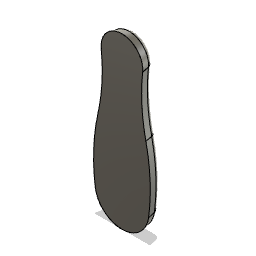
Robot_assembly (Autodesk Fusion 360 archive; units mm, degrees)
design "RBT_LINK2"
Autodesk Fusion 360 part; units mm, degrees
sketch "Sketch2" plane through (0, 0, 0) normal (0, 0, 1) x (1, 0, 0)
  arc A0 (29.8304, 196.8149) -> (35.2531, 100) centre (328.1348, 164.9639) ccw
  arc A1 (39.6352, -5.3902) -> (35.2531, 100) centre (-257.6286, 35.0361) ccw
  line L0 (0, 200) -> (0, 0) construction
  arc A2 (-35.2531, 100) -> (-29.8304, 196.8149) centre (-328.1348, 164.9639) ccw
  arc A3 (-35.2531, 100) -> (-39.6352, -5.3902) centre (257.6286, 35.0361) ccw
  arc A4 (29.8304, 196.8149) -> (-29.8304, 196.8149) centre (0, 200) ccw
  arc A5 (-39.6352, -5.3902) -> (39.6352, -5.3902) centre (0, 0) ccw
  dimension "d5" = 80
  dimension "d6" = 60
  dimension "d7" = 200
  dimension "d8" = 100
  dimension "d9" = 300
  constraint coincident L0.end A5.centre
  constraint vertical L0.end L0.start
  constraint tangent A0 A1
  constraint tangent A0 A4
  constraint tangent A1 A5
  constraint equal A0 A1
  constraint coincident L0.start A4.centre
  constraint symmetric A0.start L0 A2.end
  constraint symmetric A0.end L0 A2.start
  constraint symmetric A0 L0 A2
  constraint symmetric A1.start L0 A3.end
  constraint symmetric A1 L0 A3
  measures "d5" diameter of A5
  measures "d6" diameter of A4
  measures "d7" distance of L0.end L0.start
  measures "d8" vertical distance of L0.end A0.end
  measures "d9" radius of A0
extrude "Extrude1" add sketch "Sketch2" along normal blind 20
draft "Draft1" angle 12 neutral plane through (0, 0, 0) pull (0, 0, -1) 6 faces at (33.1008, 110.6047, 6.6667) (-29.95, 198.2683, 6.6667) (-28.3505, 153.5916, 6.6667) (-39.4474, 76.8197, 6.6667) (18.4195, -35.5067, 13.3333) (42.2994, 41.6114, 6.6667)
fillet "Fillet1" radius 10 6 edges at (-28.6043, 148.1869, 0) (-42.1125, 47.499, 0) (0, -40, 0) (42.1125, 47.499, 0) (28.6043, 148.1869, 0) (0, 230, 0)
shell "Shell4" [rolled back] inner thickness 3
ref_plane "WorkPlane1" through (0, 98.0755, 15) normal (0, 0, 1) x (1, 0, 0)
sketch "Sketch3" plane through (0, 98.0755, 15) normal (0, 0, 1) x (1, 0, 0)
  line L0 (-10, 90) -> (10, 90)
  line L1 (-10, 40) -> (10, 40)
  line L2 (-20, -20) -> (10, -20)
  line L3 (-20, -70) -> (20, -70)
  line L4 (-10, -113.3333) -> (9.4128, -113.3333)
  line L5 (-10, 20) -> (-10, -10)
  line L6 (10, 20) -> (10, -10)
  constraint horizontal L0
  constraint horizontal L1
  constraint horizontal L2
  constraint horizontal L3
  constraint horizontal L4
  constraint perpendicular L2 L5
  constraint vertical L6
web "Web1" [rolled back] thickness 2
sketch "Sketch4" plane through (0, 0, 0) normal (0, 1, 0) x (1, 0, 0)
  line L0 (-9, -3) -> (9, -15)
rib "Rib1" [rolled back] thickness 2 thickness 2

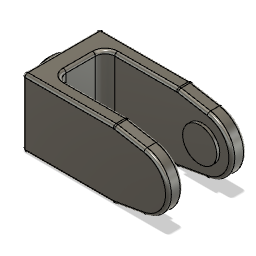
design "RBT_LINK4"
Autodesk Fusion 360 part; units mm, degrees
sketch "Sketch1" plane through (0, 0, 0) normal (0, 0, 1) x (1, 0, 0)
  line L0 (0, 0) -> (94.2683, 0)
  line L1 (94.2683, 0) -> (125.2094, 5.4558)
  arc A0 (125.2094, 5.4558) -> (125.2094, 64.5442) centre (120, 35) ccw
  line L2 (125.2094, 64.5442) -> (94.2683, 70)
  line L3 (94.2683, 70) -> (0, 70)
  line L4 (0, 70) -> (0, 0)
  dimension "d1" = 70
  dimension "d2" = 30
  dimension "d3" = 170
  dimension "d4" = 120
  constraint coincident L0.start L4.end
  constraint horizontal L0
  constraint tangent L1 A0
  constraint tangent A0 L2
  constraint horizontal L3
  constraint perpendicular L0 L4
  constraint equal L1 L2
  constraint equal L0 L3
  measures "d1" distance of L0 L3
  measures "d2" radius of A0
  measures "d3" angle of L0 L1
  measures "d4" horizontal distance of L0.start A0.centre
extrude "Extrude1" add sketch "Sketch1" along normal mid plane 80
sketch "Sketch2" plane through (0, 70, 0) normal (0, 1, 0) x (-1, 0, 0)
  line L0 (0, -40) -> (0, 40)
  line L1 (0, 40) -> (-94.2683, 40)
  line L2 (-94.2683, 40) -> (-94.2683, -40)
  line L3 (-94.2683, -40) -> (0, -40)
  line L4 (-20, -25) -> (-190, -25)
  line L5 (-190, -25) -> (-190, 25)
  line L6 (-190, 25) -> (-20, 25)
  line L7 (-20, 25) -> (-20, -25)
  dimension "d7" = 15
  dimension "d8" = 15
  dimension "d9" = 20
  dimension "d10" = 170
  constraint horizontal L4
  constraint vertical L5
  constraint horizontal L6
  constraint vertical L7
  measures "d7" distance of L3 L4
  measures "d8" distance of L1 L6
  measures "d9" distance of L0 L7
  measures "d10" distance of L5.end L6.end
extrude "Extrude2" cut sketch "Sketch2" against normal through all contours L2 L4 L5 L6 | L2 L4 L6 L7
sketch "Sketch3" plane through (0, 0, -25) normal (0, 0, 1) x (1, 0, 0)
  line L0 (20, 0) -> (94.2683, 0)
  line L1 (94.2683, 0) -> (125.2094, 5.4558)
  arc A0 (125.2094, 5.4558) -> (125.2094, 64.5442) centre (120, 35) ccw
  line L2 (125.2094, 64.5442) -> (94.2683, 70)
  line L3 (94.2683, 70) -> (20, 70)
  line L4 (20, 70) -> (20, 0)
  circle A1 centre (120, 35) radius 17.5
  dimension "d12" = 35
  constraint concentric A0 A1
  measures "d12" diameter of A1
extrude "Extrude3" add sketch "Sketch3" along normal blind 3 contours A1
mirror "Mirror1" about plane through (0, 0, 0) normal (0, 0, 1) of "Extrude3"
sketch "Sketch4" plane through (0, 0, 0) normal (-1, 0, 0) x (0, 0, 1)
  line L0 (-40, 0) -> (40, 0)
  line L1 (40, 0) -> (40, 70)
  line L2 (40, 70) -> (-40, 70)
  line L3 (-40, 70) -> (-40, 0)
  circle A0 centre (0, 35) radius 25
  line L4 (0, 35) -> (-40, 35) construction
  line L5 (0, 35) -> (0, 0) construction
  dimension "d16" = 50
  constraint coincident A0.centre L4.start
  constraint midpoint L3 L4.end
  constraint perpendicular L3 L4
  constraint coincident L5.end origin
  constraint perpendicular L0 L5
  measures "d16" diameter of A0
extrude "Extrude4" add sketch "Sketch4" along normal blind 10 contours A0
sketch "Sketch5" plane through (-10, 0, 0) normal (-1, 0, 0) x (0, 0, 1)
  circle A0 centre (0, 35) radius 25
  circle A1 centre (0, 35) radius 22
  dimension "d19" = -3
extrude "Extrude5" add sketch "Sketch5" along normal blind 3 contours A1
fillet "Fillet1" radius 10 6 edges at (20, 35, 25) (20, 35, -25) (94.2683, 70, 32.5) (94.2683, 70, -32.5) (94.2683, 0, 32.5) (94.2683, 0, -32.5)
fillet "Fillet2" radius 3 39 edges at (46.6967, 0, 40) (94.2649, 0.0381, 40) (110.1696, 2.8038, 40) (150, 35, 40) (110.1696, 67.1962, 40) (94.2649, 69.9619, 40) (46.6967, 70, 40) (46.6967, 70, -40) (94.2649, 69.9619, -40) (110.1696, 67.1962, -40) (150, 35, -40) (110.1696, 2.8038, -40) (94.2649, 0.0381, -40) (46.6967, 0, -40) (0, 70, 0) (0, 35, 40) (0, 35, -40) (0, 0, 0) (0, 44.0404, -23.3082) (22.9289, 70, 22.0711) (20, 70, 0) (22.9289, 70, -22.0711) (61.6967, 70, -25) (94.2649, 69.9619, -25) (110.1696, 67.1962, -25) (150, 35, -25) (110.1696, 2.8038, -25) (94.2649, 0.0381, -25) (61.6967, 0, -25) (22.9289, 0, -22.0711) (20, 0, 0) (22.9289, 0, 22.0711) (61.6967, 0, 25) (94.2649, 0.0381, 25) (110.1696, 2.8038, 25) (150, 35, 25) (110.1696, 67.1962, 25) (94.2649, 69.9619, 25) (61.6967, 70, 25)

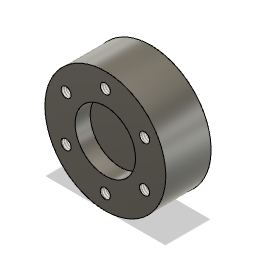
design "RBT_LINK6"
Autodesk Fusion 360 part; units mm, degrees
sketch "Sketch1" plane through (0, 0, 0) normal (0, 0, 1) x (1, 0, 0)
  circle A0 centre (0, 0) radius 20
  dimension "d1" = 40
  constraint coincident A0.centre origin
  measures "d1" diameter of A0
extrude "Extrude1" add sketch "Sketch1" along normal blind 15
sketch "Sketch2" plane through (0, 0, 15) normal (0, 0, 1) x (1, 0, 0)
  circle A0 centre (0, 0) radius 20
  circle A1 centre (0, 0) radius 10
  dimension "d4" = 20
  constraint coincident A0.centre A1.centre
  measures "d4" diameter of A1
extrude "Extrude2" cut sketch "Sketch2" against normal blind 5 contours A1
sketch "Sketch3" plane through (0, 0, 15) normal (0, 0, 1) x (1, 0, 0)
  circle A0 centre (0, 0) radius 10
  circle A1 centre (0, 0) radius 20
  point P0 (0, 15)
  dimension "d7" = 15
  constraint vertical A0.centre P0
  measures "d7" distance of A0.centre P0
hole "Hole1" at (0, 15, 15) direction (0, 0, -1) diameter 3.332 depth 8 tip angle 118
thread "Thread1" "ISO Metric profile 4.0 M4x0.7 6H"
pattern_circular "C-Pattern1" count 6 over 360 about axis through (0, 0, 1.75) along (0, 0, 1) of "Hole1"
sketch "Sketch4" plane through (0, 0, 0) normal (0, 0, -1) x (-1, 0, 0)
  circle A0 centre (0, 0) radius 20
  circle A1 centre (0, 0) radius 17.5
  dimension "d13" = 35
  constraint coincident A0.centre A1.centre
  measures "d13" diameter of A1
extrude "Extrude3" cut sketch "Sketch4" against normal blind 3 contours A1

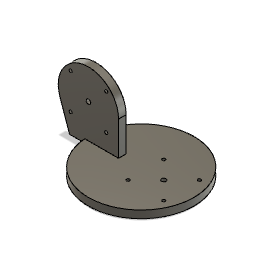
design "RBT_LINK1"
Autodesk Fusion 360 part; units mm, degrees
sketch "Sketch1" plane through (0, 0, 0) normal (0, 1, 0) x (1, 0, 0)
  circle A0 centre (0, 0) radius 70
  dimension "d1" = 140
  constraint coincident A0.centre origin
  measures "d1" diameter of A0
extrude "Extrude1" add sketch "Sketch1" along normal blind 10
sketch "Sketch2" plane through (0, 0, 0) normal (0, -1, 0) x (1, 0, 0)
  circle A0 centre (0, 0) radius 70
  circle A1 centre (0, 0) radius 65
  dimension "d4" = -5
extrude "Extrude2" add sketch "Sketch2" along normal blind 3 contours A1
sketch "Sketch3" plane through (0, 0, 0) normal (0, 0, 1) x (1, 0, 0)
  line L0 (-25, 55) -> (-25, 5)
  line L1 (-25, 5) -> (-90, 5)
  line L2 (-90, 5) -> (-102.7928, 41.8964)
  arc A0 (-25, 55) -> (-102.7928, 41.8964) centre (-65, 55) ccw
  dimension "d7" = 50
  dimension "d8" = 65
  dimension "d9" = 40
  dimension "d10" = 5
  dimension "d11" = 25
  constraint vertical L0
  constraint perpendicular L0 L1
  constraint tangent L2 A0
  constraint tangent L0 A0
  measures "d7" distance of L0.start L0.end
  measures "d8" distance of L0.end L1.end
  measures "d9" radius of A0
  measures "d10" vertical distance of origin L0.end
  measures "d11" horizontal distance of origin L0.end
extrude "Extrude3" add sketch "Sketch3" along normal mid plane 10
sketch "Sketch4" plane through (0, 10, 0) normal (0, 1, 0) x (-1, 0, 0)
  line L0 (25, 5) -> (69.8212, 5)
  arc A0 (69.8212, 5) -> (69.8212, -5) centre (0, 0) ccw
  line L1 (69.8212, -5) -> (25, -5)
  line L2 (25, -5) -> (25, 5)
  line L3 (-6.378, -23.622) -> (-53.622, -23.622)
  line L4 (-53.622, -23.622) -> (-53.622, 23.622)
  line L5 (-53.622, 23.622) -> (-6.378, 23.622)
  line L6 (-6.378, 23.622) -> (-6.378, -23.622)
  line L7 (-6.378, -23.622) -> (-53.622, 23.622) construction
  line L8 (-53.622, -23.622) -> (-6.378, 23.622) construction
  point P0 (-30, 0)
  dimension "d14" = 47.244
  dimension "d15" = 47.244
  dimension "d16" = 30
  constraint horizontal L3
  constraint perpendicular L3 L4
  constraint parallel L3 L5
  constraint parallel L4 L6
  constraint coincident L7 P0
  constraint coincident L8 P0
  constraint horizontal A0.centre P0
  measures "d14" distance of L4.end L5.end
  measures "d15" distance of L3.end L4.end
  measures "d16" distance of A0.centre P0
hole "Hole1" at (6.378, 10, 23.622) at (6.378, 10, -23.622) at (53.622, 10, -23.622) at (53.622, 10, 23.622) direction (0, -1, 0) diameter 4 depth 10 tip angle 118
hole "Hole2" at (30, 10, 0) direction (0, -1, 0) diameter 6 depth 15 tip angle 118
sketch "Sketch5" plane through (0, 0, 5) normal (0, 0, 1) x (1, 0, 0)
  line L0 (-69.8212, 10) -> (-25, 10)
  line L1 (-25, 10) -> (-25, 55)
  arc A0 (-25, 55) -> (-102.7928, 41.8964) centre (-65, 55) ccw
  line L2 (-102.7928, 41.8964) -> (-90, 5)
  line L3 (-90, 5) -> (-69.8212, 5)
  line L4 (-69.8212, 5) -> (-69.8212, 10)
  line L5 (-41.378, 78.622) -> (-88.622, 78.622)
  line L6 (-88.622, 78.622) -> (-88.622, 31.378)
  line L7 (-88.622, 31.378) -> (-41.378, 31.378)
  line L8 (-41.378, 31.378) -> (-41.378, 78.622)
  line L9 (-41.378, 78.622) -> (-88.622, 31.378) construction
  line L10 (-88.622, 78.622) -> (-41.378, 31.378) construction
  point P0 (-65, 55)
  dimension "d23" = 47.244
  dimension "d24" = 47.244
  constraint horizontal L5
  constraint perpendicular L5 L6
  constraint parallel L5 L7
  constraint parallel L6 L8
  constraint coincident L9 P0
  constraint coincident L10 P0
  constraint coincident P0 A0.centre
  measures "d23" distance of L6.end L7.end
  measures "d24" distance of L5.end L6.end
hole "Hole3" at (-88.622, 78.622, 5) at (-41.378, 78.622, 5) at (-41.378, 31.378, 5) at (-88.622, 31.378, 5) direction (0, 0, -1) diameter 4 depth 40 tip angle 118
hole "Hole4" at (-65, 55, 5) direction (0, 0, -1) diameter 6 depth 40 tip angle 118

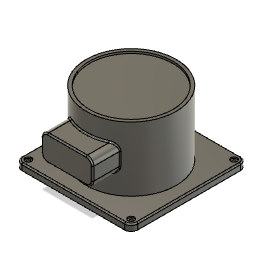
design "RBT_BASE"
Autodesk Fusion 360 part; units mm, degrees
sketch "Sketch1" plane through (0, 0, 0) normal (0, 1, 0) x (1, 0, 0)
  line L0 (90, -90) -> (-90, -90)
  line L1 (-90, -90) -> (-90, 90)
  line L2 (-90, 90) -> (90, 90)
  line L3 (90, 90) -> (90, -90)
  line L4 (90, -90) -> (-90, 90) construction
  line L5 (-90, -90) -> (90, 90) construction
  dimension "d1" = 180
  dimension "d2" = 180
  constraint horizontal L0
  constraint perpendicular L0 L1
  constraint parallel L0 L2
  constraint parallel L1 L3
  constraint coincident L4 origin
  constraint coincident L5 origin
  measures "d1" distance of L1.end L2.end
  measures "d2" distance of L0.end L1.end
extrude "Extrude1" add sketch "Sketch1" along normal blind 10
sketch "Sketch2" plane through (0, 10, 0) normal (0, 1, 0) x (-1, 0, 0)
  line L0 (-90, -90) -> (90, -90)
  line L1 (90, -90) -> (90, 90)
  line L2 (90, 90) -> (-90, 90)
  line L3 (-90, 90) -> (-90, -90)
  circle A0 centre (0, 0) radius 70
  dimension "d5" = 140
  constraint coincident A0.centre origin
  measures "d5" diameter of A0
extrude "Extrude2" add sketch "Sketch2" along normal blind 100 contours A0
sketch "Sketch3" plane through (0, 0, 0) normal (0, 0, 1) x (1, 0, 0)
  line L0 (40, 40) -> (-40, 40)
  line L1 (-40, 40) -> (-40, 80)
  line L2 (-40, 80) -> (40, 80)
  line L3 (40, 80) -> (40, 40)
  line L4 (40, 40) -> (-40, 80) construction
  line L5 (-40, 40) -> (40, 80) construction
  point P0 (0, 60)
  dimension "d8" = 80
  dimension "d9" = 40
  dimension "d10" = 60
  constraint horizontal L0
  constraint perpendicular L0 L1
  constraint parallel L0 L2
  constraint parallel L1 L3
  constraint coincident L4 P0
  constraint coincident L5 P0
  measures "d8" distance of L1.end L2.end
  measures "d9" distance of L0.end L1.end
  measures "d10" distance of origin P0
extrude "Extrude3" add sketch "Sketch3" along normal blind 100
sketch "Sketch4" plane through (0, 110, 0) normal (0, 1, 0) x (-1, 0, 0)
  circle A0 centre (0, 0) radius 70
  circle A1 centre (0, 0) radius 65
  dimension "d13" = -5
extrude "Extrude4" cut sketch "Sketch4" against normal blind 3 contours A1
sketch "Sketch5" plane through (0, 10, 0) normal (0, 1, 0) x (-1, 0, 0)
  circle A0 centre (0, 0) radius 70
  line L0 (-90, -90) -> (90, -90)
  line L1 (90, -90) -> (90, 90)
  line L2 (90, 90) -> (-90, 90)
  line L3 (-90, 90) -> (-90, -90)
  point P0 (80, -80)
  point P1 (-80, -80)
  point P2 (-80, 80)
  point P3 (80, 80)
  dimension "d16" = 10
  dimension "d17" = 10
  dimension "d18" = 10
  dimension "d19" = 10
  dimension "d20" = 10
  dimension "d21" = 10
  dimension "d22" = 10
  dimension "d23" = 10
  measures "d16" distance of L2 P3
  measures "d17" distance of L1 P3
  measures "d18" distance of L3 P2
  measures "d19" distance of L2 P2
  measures "d20" distance of L0 P1
  measures "d21" distance of L3 P1
  measures "d22" distance of L0 P0
  measures "d23" distance of L1 P0
hole "Hole1" at (-80, 10, 80) at (80, 10, 80) at (80, 10, -80) at (-80, 10, -80) direction (0, -1, 0) diameter 5 depth 10 tip angle 118 counterbore diameter 10 counterbore depth 2
fillet "Fillet1" radius 10 8 edges at (-90, 5, 90) (90, 5, 90) (90, 5, -90) (-90, 5, -90) (-40, 80, 78.7228) (-40, 40, 78.7228) (40, 80, 78.7228) (40, 40, 78.7228)
fillet "Fillet2" radius 2 24 edges at (87.0711, 10, -87.0711) (0, 10, -90) (-87.0711, 10, -87.0711) (-90, 10, 0) (-87.0711, 10, 87.0711) (0, 10, 90) (87.0711, 10, 87.0711) (90, 10, 0) (36.9012, 77.2363, 59.4835) (40, 60, 57.4456) (36.9012, 42.7637, 59.4835) (0, 40, 70) (-36.9012, 42.7637, 59.4835) (-40, 60, 57.4456) (-36.9012, 77.2363, 59.4835) (0, 80, 70) (-37.0711, 77.0711, 100) (-40, 60, 100) (-37.0711, 42.9289, 100) (0, 40, 100) (37.0711, 42.9289, 100) (40, 60, 100) (37.0711, 77.0711, 100) (0, 80, 100)

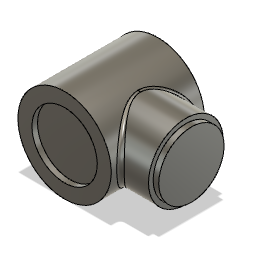
design "RBT_LINK5"
Autodesk Fusion 360 part; units mm, degrees
sketch "Sketch1" plane through (0, 0, 0) normal (0, 0, 1) x (1, 0, 0)
  circle A0 centre (0, 0) radius 25
  dimension "d1" = 50
  constraint coincident A0.centre origin
  measures "d1" diameter of A0
extrude "Extrude1" add sketch "Sketch1" along normal mid plane 50
sketch "Sketch2" plane through (0, 0, 25) normal (0, 0, 1) x (1, 0, 0)
  circle A0 centre (0, 0) radius 25
  circle A1 centre (0, 0) radius 17.5
  dimension "d4" = 35
  constraint concentric A0 A1
  measures "d4" diameter of A1
extrude "Extrude2" cut sketch "Sketch2" against normal blind 3 contours A1
mirror "Mirror1" about plane through (0, 0, 0) normal (0, 0, 1) of "Extrude2"
sketch "Sketch3" plane through (0, 0, 0) normal (1, 0, 0) x (0, 0, -1)
  circle A0 centre (0, 0) radius 20
  dimension "d8" = 40
  constraint coincident A0.centre origin
  measures "d8" diameter of A0
extrude "Extrude3" add sketch "Sketch3" along normal blind 40
sketch "Sketch4" plane through (40, 0, 0) normal (1, 0, 0) x (0, 0, -1)
  circle A0 centre (0, 0) radius 20
  circle A1 centre (0, 0) radius 17.5
  dimension "d11" = 35
  constraint concentric A0 A1
  measures "d11" diameter of A1
extrude "Extrude4" add sketch "Sketch4" along normal blind 3 contours A1
fillet "Fillet1" radius 2 1 edges at (15, -20, 0)

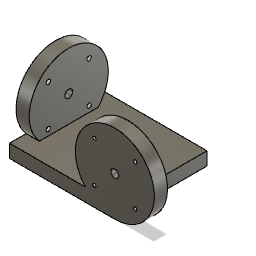
design "RBT_LINK3"
Autodesk Fusion 360 part; units mm, degrees
sketch "Sketch1" plane through (0, 0, 0) normal (0, 0, 1) x (1, 0, 0)
  circle A0 centre (0, 0) radius 30
  dimension "d1" = 60
  constraint coincident A0.centre origin
  measures "d1" diameter of A0
extrude "Extrude1" add sketch "Sketch1" along normal blind 10
sketch "Sketch2" plane through (0, 0, 10) normal (0, 0, 1) x (1, 0, 0)
  circle A0 centre (0, 0) radius 30
  line L0 (0, -30) -> (-80, -30)
  line L1 (-80, -30) -> (-80, -20)
  line L2 (-80, -20) -> (0, -20)
  line L3 (0, -20) -> (0, -30)
  dimension "d4" = 80
  dimension "d5" = 10
  constraint horizontal L0
  constraint vertical L1
  constraint horizontal L2
  constraint vertical L3
  constraint coincident A0 L0.start
  constraint vertical A0.centre L0.start
  measures "d4" distance of L0.start L0.end
  measures "d5" distance of L0.start L2.end
extrude "Extrude2" add sketch "Sketch2" against normal blind 70 contours A0 L0 L1 L2 | A0 L2 L3 picked at (-1.3972, -26.5686)
sketch "Sketch3" plane through (-80, 0, 0) normal (-1, 0, 0) x (0, 0, 1)
  line L0 (10, -30) -> (10, -20)
  line L1 (10, -20) -> (-60, -20)
  line L2 (-60, -20) -> (-60, -30)
  line L3 (-60, -30) -> (10, -30)
  circle A0 centre (-25, 0) radius 30
  line L4 (-25, -30) -> (-25, 0) construction
  dimension "d8" = 60
  constraint horizontal origin A0.centre
  constraint midpoint L3 L4.start
  constraint coincident A0.centre L4.end
  constraint vertical L4
  measures "d8" diameter of A0
extrude "Extrude3" add sketch "Sketch3" against normal blind 10 contours L1 A0 picked at (-32.7403, 15.1228)
sketch "Sketch4" plane through (0, 0, 0) normal (0, 0, -1) x (-1, 0, 0)
  line L0 (0, -30) -> (0, -20)
  line L1 (0, -20) -> (22.3607, -20)
  arc A0 (22.3607, -20) -> (0, -30) centre (0, 0) ccw
  line L2 (15.5, -15.5) -> (-15.5, -15.5)
  line L3 (-15.5, -15.5) -> (-15.5, 15.5)
  line L4 (-15.5, 15.5) -> (15.5, 15.5)
  line L5 (15.5, 15.5) -> (15.5, -15.5)
  line L6 (15.5, -15.5) -> (-15.5, 15.5) construction
  line L7 (-15.5, -15.5) -> (15.5, 15.5) construction
  dimension "d11" = 31
  dimension "d12" = 31
  constraint horizontal L2
  constraint perpendicular L2 L3
  constraint parallel L2 L4
  constraint parallel L3 L5
  constraint coincident L6 A0.centre
  constraint coincident L7 A0.centre
  constraint coincident A0.centre origin
  measures "d11" distance of L3.end L4.end
  measures "d12" distance of L2.end L3.end
hole "Hole1" at (-15.5, 15.5, 0) at (15.5, 15.5, 0) at (15.5, -15.5, 0) at (-15.5, -15.5, 0) direction (0, 0, 1) diameter 2.529 depth 10 tip angle 118
thread "Thread1" "ISO Metric profile 3.0 M3x0.5 6H"
hole "Hole2" at (0, 0, 0) direction (0, 0, 1) diameter 6 depth 10 tip angle 118
sketch "Sketch5" plane through (-80, 0, 0) normal (-1, 0, 0) x (0, 0, 1)
  line L0 (10, -30) -> (10, -20)
  line L1 (10, -20) -> (-2.6393, -20)
  arc A0 (-2.6393, -20) -> (-47.3607, -20) centre (-25, 0) ccw
  line L2 (-47.3607, -20) -> (-60, -20)
  line L3 (-60, -20) -> (-60, -30)
  line L4 (-60, -30) -> (10, -30)
  line L5 (-40.5, 15.5) -> (-9.5, 15.5)
  line L6 (-9.5, 15.5) -> (-9.5, -15.5)
  line L7 (-9.5, -15.5) -> (-40.5, -15.5)
  line L8 (-40.5, -15.5) -> (-40.5, 15.5)
  line L9 (-40.5, 15.5) -> (-9.5, -15.5) construction
  line L10 (-9.5, 15.5) -> (-40.5, -15.5) construction
  point P0 (-25, 0)
  dimension "d19" = 31
  dimension "d20" = 31
  constraint horizontal L5
  constraint perpendicular L5 L6
  constraint parallel L5 L7
  constraint parallel L6 L8
  constraint coincident L9 P0
  constraint coincident L10 P0
  constraint coincident P0 A0.centre
  measures "d19" distance of L6.end L7.end
  measures "d20" distance of L5.end L6.end
hole "Hole3" at (-80, 15.5, -40.5) at (-80, 15.5, -9.5) at (-80, -15.5, -40.5) at (-80, -15.5, -9.5) direction (1, 0, 0) diameter 3.332 depth 40 tip angle 118
thread "Thread2" "ISO Metric profile 4.0 M4x0.7 6H"
hole "Hole4" at (-80, 0, -25) direction (1, 0, 0) diameter 6 depth 40 tip angle 118
